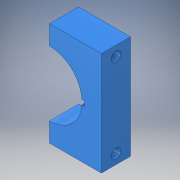
# Autodesk Inventor part: gripperBracketB
Saved by Autodesk Inventor 2018.2 (Build 222227000, 227)
## iProperties
Created: 2018-02-13
Part Number: gripperBracketB
Material: Aluminum 6061
Document SubType Name: Modeling
Designer: steele
Density: 2.7 g/cm^3
Appearance: Cyan
Author: steele
Autodesk Inventor part; units mm, degrees
ref_plane "YZ Plane" through (0, 0, 0) normal (1, 0, 0) x (0, 1, 0)
ref_plane "XZ Plane" through (0, 0, 0) normal (0, 1, 0) x (-1, 0, 0)
ref_plane "XY Plane" through (0, 0, 0) normal (0, 0, 1) x (1, 0, 0)
sketch "Sketch1" plane through (0, 0, 0) normal (0, 0, 1) x (1, 0, 0)
  arc A0 (21.2132, 1.5875) -> (21.2132, -1.5875) centre (0, 0) ccw
  arc A1 (0, 33.9725) -> (-33.9725, 0) centre (0, 0) ccw
  line L0 (0, -33.9725) -> (-33.9725, -33.9725)
  line L1 (-33.9725, 0) -> (-33.9725, -33.9725)
  line L2 (0, 33.9725) -> (33.9725, 33.9725)
  line L3 (0, -33.9725) -> (33.9725, -33.9725)
  line L4 (33.9725, 0) -> (33.9725, -33.9725)
  line L5 (33.9725, 0) -> (33.9725, 33.9725)
  line L6 (0, 0) -> (24.13, 0) construction
  line L7 (21.2132, 1.5875) -> (22.8007, 1.5875)
  line L8 (22.8007, 1.5875) -> (22.8007, -1.5875)
  line L9 (22.8007, -1.5875) -> (21.2132, -1.5875)
  dimension "d0" = 42.545
  dimension "d1" = 67.945
  dimension "d22" = 1.5875
  dimension "d23" = 1.5875
  dimension "d24" = 1.5875
  constraints: 20 end point, 5 horizontal, 5 perpendicular, 5 tangent, 4 point on circle, 2 centre point, 2 coincident
  measures "d0" diameter of A0
  measures "d1" diameter of A1
  measures "d22" distance between parallel lines of L6 L7
  measures "d23" distance between parallel lines of L6 L9
  measures "d24" distance from line of L8 L7.start
extrude "Extrusion1" add sketch "Sketch1" along normal mid plane 19.05
sketch "Sketch2" plane through (-33.9725, -33.9725, 9.525) normal (-1, 0, 0) x (0, 0, 1)
  line L0 (0, 0) -> (-19.05, 0) construction
  line L1 (-9.525, 0) -> (-9.525, 33.9725) construction
  point P0 (-9.525, 10.16)
  dimension "d4" = 10.16
  constraints: 2 end point, 1 midpoint, 1 point on line, 1 vertical
  measures "d4" distance from line of point (-9.525, 10.16) L0
hole "Hole1" at (-33.9725, -23.8125, 0) direction (1, 0, 0) diameter 4.9784 depth 31.75 tip angle 118 thread size "1/4-20 UNC" class "2B" standard "ANSI Unified Screw Threads"
sketch "Sketch3" plane through (33.9725, -33.9725, 9.525) normal (1, 0, 0) x (0, 0, -1)
  line L0 (0, 67.945) -> (19.05, 67.945) construction
  line L1 (9.525, 67.945) -> (9.525, 0) construction
  line L2 (0, 0) -> (19.05, 0) construction
  point P0 (9.525, 33.9725)
  point P1 (9.525, 61.595)
  point P2 (9.525, 6.35)
  dimension "d13" = 6.35
  dimension "d14" = 6.35
  constraints: 2 end point, 2 midpoint, 2 point on line
  measures "d13" distance from line of point (9.525, 61.595) L0
  measures "d14" distance from line of point (9.525, 6.35) L2
split "Split1" plane through (0, 0, 0) removes the side toward (-1, 0, 0)
hole "Hole2" at (33.9725, 27.6225, 0) at (33.9725, -27.6225, 0) direction (-1, 0, 0) diameter 6.35 end through all
equation "\"d0\" = pipeDiameter"
equation "\"d1\" = pipeDiameter + 2 * outerRadius"
equation "\"d2\" = width"
equation "\"pipeDiameter\" = 42.545"
equation "\"outerRadius\" = 12.7"
equation "\"width\" = 19.05"
body "Solid1"
